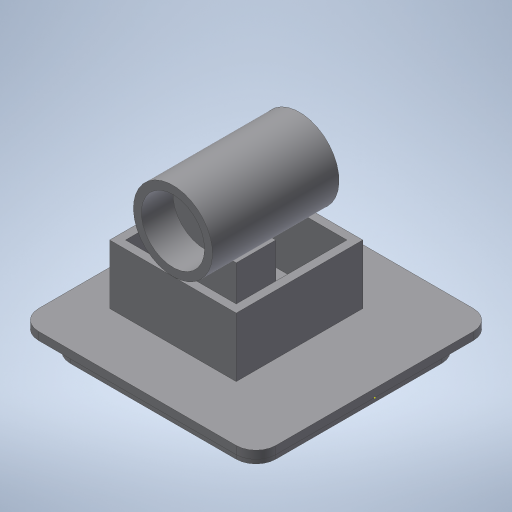
# Autodesk Inventor part: Pieza 3.1 final
Saved by Autodesk Inventor 2023.1 (Build 271208000, 208)
## iProperties
Created: 2022-10-20
Part Number: Pieza 3.1 final
Material: Generic
Document SubType Name: Modeling
Designer: User
Density: 1 g/cm^3
Appearance: Default
Author: User
Autodesk Inventor part; units mm, degrees
ref_plane "YZ Plane" through (0, 0, 0) normal (1, 0, 0) x (0, 1, 0)
ref_plane "XZ Plane" through (0, 0, 0) normal (0, 1, 0) x (-1, 0, 0)
ref_plane "XY Plane" through (0, 0, 0) normal (0, 0, 1) x (1, 0, 0)
sketch "Sketch1" plane through (0, 0, 0) normal (0, 1, 0) x (-1, 0, 0)
  line L0 (0, 0) -> (60, 0)
  line L1 (60, 0) -> (60, -60)
  line L2 (60, -60) -> (0, -60)
  line L3 (0, -60) -> (0, 0)
  dimension "d0" = 60
  dimension "d1" = 60
  constraints: 8 end point, 2 parallel, 1 horizontal, 1 perpendicular
  measures "d0" distance of L1.end L2.end
  measures "d1" distance of L0.end L1.end
extrude "Extrusion1" add sketch "Sketch1" along normal blind 2
sketch "Sketch2" plane through (0, 0, 0) normal (0, -1, 0) x (1, 0, 0)
  line L0 (0, -60) -> (-60, -60) projected
  line L1 (0, 0) -> (0, -60) projected
  line L2 (-60, 0) -> (0, 0) projected
  line L3 (-60, -60) -> (-60, 0) projected
  line L4 (-6, -6) -> (-6, -54)
  line L5 (-6, -54) -> (-54, -54)
  line L6 (-54, -54) -> (-54, -6)
  line L7 (-54, -6) -> (-6, -6)
  line L8 (-4, -4) -> (-4, -56)
  line L9 (-4, -56) -> (-56, -56)
  line L10 (-56, -56) -> (-56, -4)
  line L11 (-56, -4) -> (-4, -4)
  dimension "d4" = 6
  dimension "d5" = 4
  constraints: 16 end point, 6 other
  measures "d4" distance between parallel lines of L2 L7
  measures "d5" distance between parallel lines of L2 L11
extrude "Extrusion2" add sketch "Sketch2" along normal blind 5 contours L8 L9 L10 L11
sketch "Sketch10" plane through (0, 2, 0) normal (0, 1, 0) x (1, 0, 0)
  line L0 (0, 60) -> (-60, 60) projected
  line L1 (-60, 60) -> (-60, 0) projected
  line L2 (-60, 0) -> (0, 0) projected
  line L3 (0, 0) -> (0, 60) projected
sketch "Sketch11" plane through (0, 2, 0) normal (0, 1, 0) x (1, 0, 0)
  line L0 (0, 60) -> (-60, 60) projected
  line L1 (-60, 60) -> (-60, 0) projected
  line L2 (-60, 0) -> (0, 0) projected
  line L3 (0, 0) -> (0, 60) projected
  line L4 (0, 60) -> (-60, 60) construction
  line L5 (0, 60) -> (-60, 0) construction
  line L6 (-60, 60) -> (-60, 0) projected
  line L7 (-60, 30) -> (-51, 30)
  line L8 (-51, 30) -> (-51, 46) construction
  line L9 (-51, 46) -> (-19, 46) construction
  line L10 (-19, 46) -> (-19, 14) construction
  line L11 (-19, 14) -> (-51, 14) construction
  line L12 (-51, 14) -> (-51, 46) construction
  line L13 (-51, 46) -> (-19, 46)
  line L14 (-19, 46) -> (-19, 14)
  line L15 (-19, 14) -> (-51, 14)
  line L16 (-51, 14) -> (-51, 46)
  line L17 (-51, 30) -> (-49, 30) construction
  line L18 (-49, 30) -> (-49, 44) construction
  line L19 (-49, 44) -> (-21, 44) construction
  line L20 (-21, 44) -> (-21, 16) construction
  line L21 (-21, 16) -> (-49, 16) construction
  line L22 (-49, 16) -> (-49, 44) construction
  line L23 (-49, 44) -> (-21, 44)
  line L24 (-21, 44) -> (-21, 16)
  line L25 (-21, 16) -> (-49, 16)
  line L26 (-49, 16) -> (-49, 44)
  dimension "d49" = 9
  dimension "d50" = 16
  dimension "d51" = 32
  dimension "d52" = 32
  dimension "d53" = 2
  dimension "d54" = 14
  dimension "d55" = 28
  dimension "d56" = 28
  dimension "d57" = 28
  dimension "d58" = 28
  constraints: 42 end point, 8 parallel, 6 horizontal, 4 perpendicular, 2 vertical, 1 midpoint
  measures "d49" distance of L7.start L7.end
  measures "d50" distance of L7.end L8.end
  measures "d51" distance of L10.end L11.end
  measures "d52" distance of L9.end L10.end
  measures "d53" distance of L7.end L17.end
  measures "d54" distance of L17.end L18.end
  measures "d55" distance of L20.end L21.end
  measures "d56" distance of L19.end L20.end
  measures "d57" distance of L20.end L25.end
  measures "d58" distance of L23.end L20.end
extrude "Extrusion9" add sketch "Sketch11" along normal blind 15 contours L13 L14 L15 L16
sketch "Sketch12" plane through (0, 2, 0) normal (0, 1, 0) x (1, 0, 0)
  line L0 (-49, 44) -> (-49, 16) projected
  line L1 (-49, 16) -> (-21, 16) projected
  line L2 (-21, 16) -> (-21, 44) projected
  line L3 (-21, 44) -> (-49, 44) projected
  line L4 (-49, 16) -> (-49, 44) construction
  line L5 (-49, 44) -> (-21, 44) construction
  line L6 (-49, 16) -> (-21, 44) construction
  line L7 (-21, 44) -> (-49, 44) construction
  line L8 (-49, 44) -> (-21, 16) construction
  line L9 (-40, 25) -> (-30, 25) construction
  line L10 (-30, 25) -> (-30, 35) construction
  line L11 (-30, 35) -> (-40, 35) construction
  line L12 (-40, 35) -> (-40, 25) construction
  line L13 (-40, 25) -> (-30, 35) construction
  line L14 (-30, 25) -> (-40, 35) construction
  line L15 (-40, 25) -> (-30, 25)
  line L16 (-30, 25) -> (-30, 35)
  line L17 (-30, 35) -> (-40, 35)
  line L18 (-40, 35) -> (-40, 25)
  line L19 (-40, 25) -> (-30, 35) construction
  line L20 (-30, 25) -> (-40, 35) construction
  point P0 (0, 0)
  point P1 (-35, 30)
  dimension "d61" = 10
  dimension "d62" = 10
  dimension "d63" = 10
  dimension "d64" = 10
  constraints: 30 end point, 5 equal length, 5 midpoint, 3 perpendicular, 2 horizontal
  measures "d61" distance of L11.end L10.end
  measures "d62" distance of L10.end L9.end
  measures "d63" distance of L17.end L10.end
  measures "d64" distance of L10.end L15.end
extrude "Extrusion10" add sketch "Sketch12" along normal blind 15 contours L18 L17 L16 L15
ref_plane "Work Plane3" through (-40, 2, -30) normal (0, 0, 1) x (1, 0, 0)
sketch "Sketch13" plane through (-40, 2, -30) normal (0, 0, 1) x (1, 0, 0)
  point P0 (40, -2)
sketch "Sketch14" plane through (-40, 2, -30) normal (0, 0, 1) x (1, 0, 0)
  line L0 (0, 0) -> (0, 15) projected
  line L1 (0, 15) -> (5, 15)
  line L2 (5, 15) -> (5, 25)
  circle A0 centre (5, 25) radius 10
  point P0 (40, -2)
  dimension "d68" = 5
  dimension "d69" = 10
  dimension "d70" = 20
  constraints: 4 end point, 1 centre point, 1 coincident, 1 horizontal, 1 perpendicular
  measures "d68" distance of L0.end L1.end
  measures "d69" distance of L1.end L2.end
  measures "d70" diameter of A0
extrude "Extrusion11" add sketch "Sketch14" along normal mid plane 32
sketch "Sketch15" plane through (-35, 27, -46) normal (0, 0, -1) x (-1, 0, 0)
  circle A0 centre (0, 0) radius 10 projected
  circle A1 centre (0, 0) radius 8
  point P0 (-35, -27)
  point P1 (0, -10)
  dimension "d73" = 2
  constraints: 1 centre point, 1 vertical alignment
extrude "Extrusion12" cut sketch "Sketch15" against normal blind 8 contours A1
sketch "Sketch16" plane through (-35, 27, -14) normal (0, 0, 1) x (1, 0, 0)
  circle A0 centre (0, 0) radius 8 projected
  circle A1 centre (0, 0) radius 10 projected
  circle A2 centre (0, 0) radius 8
  point P0 (35, -27)
  point P1 (0, -10)
  dimension "d76" = 2
  constraints: 1 centre point, 1 vertical alignment
extrude "Extrusion13" cut sketch "Sketch16" against normal blind 8 contours A0
sketch "Sketch17" plane through (0, 2, 0) normal (0, 1, 0) x (1, 0, 0)
  line L0 (-35, 16) -> (-49, 16) construction
  line L1 (-21, 44) -> (-21, 16) construction
  line L2 (-49, 16) -> (-21, 44) construction
  line L3 (-21, 44) -> (-49, 44) construction
  line L4 (-49, 16) -> (-21, 16) construction
  line L5 (-49, 44) -> (-21, 16) construction
  line L6 (-30, 25) -> (-40, 25) construction
  line L7 (-40, 25) -> (-40, 35) construction
  line L8 (-40, 35) -> (-30, 35) construction
  line L9 (-30, 35) -> (-30, 25) construction
  line L10 (-49, 44) -> (-49, 16) construction
  line L11 (-49, 16) -> (-21, 16) construction
  line L12 (-21, 16) -> (-21, 44) construction
  line L13 (-21, 44) -> (-49, 44) construction
  line L14 (-49, 16) -> (-44.5, 16) construction
  line L15 (-44.5, 16) -> (-44.5, 44) construction
  circle A0 centre (-44.5, 20.5) radius 3.5
  circle A1 centre (-44.5, 39.5) radius 3.5
  point P0 (0, 0)
  dimension "d79" = 4.5
  dimension "d80" = 7
  dimension "d81" = 7
  constraints: 10 end point, 6 point on line, 3 perpendicular, 2 centre point
  measures "d79" distance of L10.end L14.end
  measures "d80" diameter of A0
  measures "d81" diameter of A1
extrude "Extrusion14" cut sketch "Sketch17" against normal blind 8
fillet "Fillet2" radius 5 12 edges at (-4, -2.5, -56) (0, 1, -60) (-6, -2.5, -54) (0, 1, 0) (-4, -2.5, -4) (-6, -2.5, -6) (-56, -2.5, -4) (-60, 1, 0) (-54, -2.5, -6) (-56, -2.5, -56) (-60, 1, -60) (-54, -2.5, -54)
sketch "Sketch4" plane through (0, 2, 0) normal (0, 1, 0) x (1, 0, 0)
  line L0 (0, 60) -> (-60, 60) construction
  line L1 (-60, 60) -> (-60, 0) construction
  line L2 (-60, 0) -> (0, 0) construction
  line L3 (0, 0) -> (0, 60) construction
  line L4 (-60, 60) -> (-60, 0) construction
  line L5 (0, 60) -> (-60, 60) construction
  line L6 (-60, 0) -> (0, 60) construction
  line L7 (0, 60) -> (-60, 60) construction
  line L8 (-60, 0) -> (0, 0) construction
  line L9 (0, 0) -> (-60, 60) construction
  line L10 (-46, 46) -> (-14, 46)
  line L11 (-14, 46) -> (-14, 14)
  line L12 (-14, 14) -> (-46, 14)
  line L13 (-46, 14) -> (-46, 46)
  line L14 (-46, 46) -> (-14, 14) construction
  line L15 (-14, 46) -> (-46, 14) construction
  line L16 (-44, 44) -> (-16, 44)
  line L17 (-16, 44) -> (-16, 16)
  line L18 (-16, 16) -> (-44, 16)
  line L19 (-44, 16) -> (-44, 44)
  line L20 (-44, 44) -> (-16, 16) construction
  line L21 (-16, 44) -> (-44, 16) construction
  line L22 (-60, 60) -> (-60, 30)
  line L23 (-60, 30) -> (-51, 30)
  line L24 (-51, 30) -> (-51, 46)
  line L25 (-51, 46) -> (-51, 14)
  line L26 (-51, 46) -> (-19, 46)
  line L27 (-19, 46) -> (-19, 14)
  line L28 (-19, 14) -> (-51, 14)
  line L29 (-51, 14) -> (-51, 46)
  line L30 (-51, 30) -> (-49, 30)
  line L31 (-49, 44) -> (-21, 44)
  line L32 (-21, 44) -> (-21, 16)
  line L33 (-21, 16) -> (-49, 16)
  line L34 (-49, 16) -> (-49, 44)
  point P0 (-30, 30)
  dimension "d15" = 32
  dimension "d16" = 32
  dimension "d17" = 28
  dimension "d18" = 28
  dimension "d43" = 9
  dimension "d44" = 16
  dimension "d45" = 32
  dimension "d46" = 32
  dimension "d47" = 2
  dimension "d48" = 28
  constraints: 56 end point, 9 equal length, 6 midpoint, 6 perpendicular, 5 horizontal, 3 point on line, 1 vertical
  measures "d15" distance of L11.end L12.end
  measures "d16" distance of L10.end L11.end
  measures "d17" distance of L17.end L18.end
  measures "d18" distance of L16.end L17.end
  measures "d43" distance of L22.end L23.end
  measures "d44" distance of L23.end L24.end
  measures "d45" distance of L24.end L25.end
  measures "d46" distance of L27.end L28.end
  measures "d47" distance of L23.end L30.end
  measures "d48" distance of L32.end L33.end
sketch "Sketch5" plane through (0, 2, 0) normal (0, 1, 0) x (1, 0, 0)
  line L0 (-44, 44) -> (-44, 16) projected
  line L1 (-44, 16) -> (-16, 16) projected
  line L2 (-16, 16) -> (-16, 44) projected
  line L3 (-16, 44) -> (-44, 44) projected
  line L4 (-60, 60) -> (-60, 0) construction
  line L5 (0, 0) -> (0, 60) construction
  line L6 (-60, 60) -> (0, 0) construction
  line L7 (0, 0) -> (0, 60) construction
  line L8 (-60, 0) -> (0, 0) construction
  line L9 (0, 60) -> (-60, 0) construction
  line L10 (-35, 35) -> (-25, 35)
  line L11 (-25, 35) -> (-25, 25)
  line L12 (-25, 25) -> (-35, 25)
  line L13 (-35, 25) -> (-35, 35)
  line L14 (-35, 35) -> (-25, 25) construction
  line L15 (-25, 35) -> (-35, 25) construction
  point P0 (-30, 30)
  dimension "d21" = 10
  dimension "d22" = 10
  constraints: 18 end point, 3 equal length, 3 midpoint, 2 perpendicular, 1 horizontal
  measures "d21" distance of L11.end L12.end
  measures "d22" distance of L10.end L11.end
sketch "Sketch6" plane through (-35, 2, -30) normal (0, 0, 1) x (1, 0, 0)
  line L0 (10, 0) -> (10, 15) construction
  line L1 (10, 15) -> (5, 15) construction
  line L2 (10, 15) -> (0, 15) construction
  line L3 (5, 15) -> (5, 25)
  circle A0 centre (5, 25) radius 10
  point P0 (35, -2)
  dimension "d26" = 5
  dimension "d27" = 10
  dimension "d28" = 20
  constraints: 4 end point, 1 centre point, 1 coincident, 1 midpoint, 1 vertical
  measures "d26" distance of L0.end L1.end
  measures "d27" distance of L1.end L3.end
  measures "d28" diameter of A0
sketch "Sketch7" plane through (-30, 27, -46) normal (0, 0, -1) x (-1, 0, 0)
  circle A0 centre (0, 0) radius 10 projected
  circle A1 centre (0, 0) radius 8
  point P0 (-30, -27)
  point P1 (0, -10)
  dimension "d31" = 2
  constraints: 1 centre point, 1 vertical alignment
sketch "Sketch8" plane through (-30, 27, -14) normal (0, 0, 1) x (1, 0, 0)
  circle A0 centre (0, 0) radius 10 projected
  circle A1 centre (0, 0) radius 8
  point P0 (30, -27)
  point P1 (0, -10)
  dimension "d34" = 2
  constraints: 1 centre point, 1 vertical alignment
body "Solid1"
